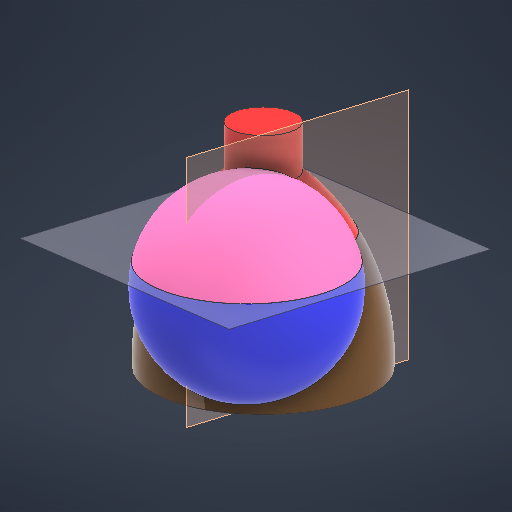
# Autodesk Inventor part: Друк 521703 lab2
Saved by Autodesk Inventor 2026 (Build 300175000, 175)
## iProperties
Created: 2025-10-21
Part Number: Друк 521703 lab2
Material: Типовые
Document SubType Name: Modeling
Designer: stud517
Density: 1 g/cm^3
Appearance: По умолчанию
Mass: 637.598 g
Surface Area: 577.422 cm^2
Volume: 637.598 cm^3
Author: stud517
Autodesk Inventor part; units mm, degrees
ref_plane "XY Plane" through (0, 0, 0) normal (0, 0, 1) x (1, 0, 0)
sketch "Эскиз1" plane through (0, 0, 0) normal (1, 0, 0) x (0, 1, 0)
  line L0 (0, 0) -> (0, -50)
  line L1 (80, 0) -> (80, -15)
  line L2 (80, -15) -> (100, -15)
  line L3 (100, -15) -> (100, 0)
  line L4 (0, 0) -> (80, 0)
  arc A0 (0, -50) -> (80, -15) centre (3.9402, 49.9223) ccw
  line L5 (100, 0) -> (80, 0)
  dimension "d0" = 50
  dimension "d2" = 15
  dimension "d3" = 20
  dimension "d4" = 100
  constraints: 12 end point, 3 horizontal, 3 vertical, 2 point on circle, 1 centre point
  measures "d0" distance of L0.start L0.end
  measures "d2" distance of L1.start L1.end
  measures "d3" distance of L1.end L2.end
  measures "d4" radius of A0
revolve "Вращение1" add sketch "Эскиз1" angle 360 about axis through (0, 0, 0) along (0, 1, 0)
ref_plane "РабПлоскость1" through (20, 0, 0) normal (1, 0, 0) x (0, 1, 0)
sketch "Эскиз2" plane through (20, 0, 0) normal (1, 0, 0) x (0, 1, 0)
  line L0 (80, -15) -> (80, 15) projected
  line L1 (0, -50) -> (0, 50) projected
  line L2 (0, 25) -> (45, 25)
  arc A0 (0, 25) -> (90, 25) centre (45, 25) ccw
  line L3 (0, 25) -> (90, 25)
  point P0 (0, 0)
  constraints: 4 end point, 2 point on circle, 2 point on line, 1 centre point, 1 coincident, 1 horizontal
revolve "Вращение2" add sketch "Эскиз2" angle 360 about axis through (20, 0, 25) along (0, 1, 0)
ref_plane "РабПлоскость2" through (0, 55, 0) normal (0, 1, 0) x (-1, 0, 0)
split_face "Разделение1"
sketch "Эскиз3" plane through (0, 55, 0) normal (0, 1, 0) x (-1, 0, 0)
  point P0 (0, 0)
sketch "Эскиз4" plane through (0, 55, 0) normal (0, 1, 0) x (-1, 0, 0)
  arc A0 (-31.6368, -17.3035) -> (23.8261, 27.0668) centre (0, 0) ccw projected
  arc A1 (23.8261, 27.0668) -> (-31.6368, -17.3035) centre (-20, 25) ccw projected
  arc A2 (-31.6368, -17.3035) -> (23.8261, 27.0668) centre (0, 0) ccw projected
  arc A3 (-14.7381, -2.7905) -> (5.9577, 13.7661) centre (0, 0) ccw projected
  line L0 (54.1182, 75.3546) -> (54.1182, -54.3405)
  line L1 (54.1182, -54.3405) -> (-69.6139, -54.3405)
  line L2 (-69.6139, -54.3405) -> (-69.6139, 75.3546)
  line L3 (-69.6139, 75.3546) -> (54.1182, 75.3546)
  point P0 (23.8261, 27.0668)
  point P1 (-31.6368, -17.3035)
  constraints: 8 end point, 3 perpendicular, 1 vertical, 5 other
extrude "Выдавливание1" add sketch "Эскиз4" along normal blind 0.1 separate body
